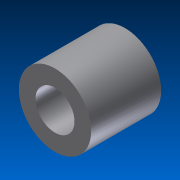
# Autodesk Inventor part: separador 4.2mm
Saved by Autodesk Inventor 2012 (Build 160160000, 160)
## iProperties
Created: 2014-01-03
Part Number: separador 4.2mm
Material: Default
Document SubType Name: Modeling
Designer: Thinkpad
Mass: 0.0440703 g
Surface Area: 1.09126 cm^2
Volume: 0.0440703 cm^3
Density: 1 g/cm^3
Author: Thinkpad
Autodesk Inventor part; units mm, degrees
ref_plane "YZ Plane" through (0, 0, 0) normal (1, 0, 0) x (0, 1, 0)
ref_plane "XZ Plane" through (0, 0, 0) normal (0, 1, 0) x (-1, 0, 0)
ref_plane "XY Plane" through (0, 0, 0) normal (0, 0, 1) x (1, 0, 0)
sketch "Sketch1" plane through (0, 0, 0) normal (0, 0, 1) x (1, 0, 0)
  circle A0 centre (0, 0) radius 1.17
  circle A1 centre (0, 0) radius 2.17
  dimension "d0" = 2.34
  dimension "d1" = 4.34
  constraints: 2 centre point, 2 coincident
  measures "d0" diameter of A0
  measures "d1" diameter of A1
extrude "Extrusion1" add sketch "Sketch1" against normal blind 4.2
body "Solid1"
